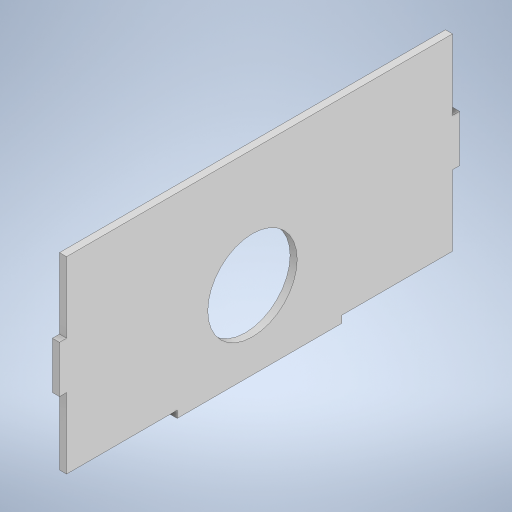
# Autodesk Inventor part: Kanan Kipas
Saved by Autodesk Inventor 2024 (Build 280153000, 153)
## iProperties
Created: 2023-08-09
Part Number: Kanan Kipas
Material: Generic
Document SubType Name: Modeling
Designer: Asus
Density: 1 g/cm^3
Appearance: Default
Author: Asus
Autodesk Inventor part; units mm, degrees
ref_plane "YZ Plane" through (0, 0, 0) normal (1, 0, 0) x (0, 1, 0)
ref_plane "XZ Plane" through (0, 0, 0) normal (0, 1, 0) x (-1, 0, 0)
ref_plane "XY Plane" through (0, 0, 0) normal (0, 0, 1) x (1, 0, 0)
sketch "Sketch2" plane through (0, 0, 0) normal (1, 0, 0) x (0, 1, 0)
  line L0 (0, 0) -> (3, 0) construction
  line L1 (3, 0) -> (3, -3)
  line L2 (3, -3) -> (3, -50)
  line L3 (3, -50) -> (0, -50)
  line L4 (0, -50) -> (0, -120)
  line L5 (0, -120) -> (3, -120)
  line L6 (3, -120) -> (3, -170)
  line L7 (33, -170) -> (33, -167)
  line L8 (53, -167) -> (53, -170)
  line L9 (53, 0) -> (53, -3)
  line L10 (33, -3) -> (33, 0)
  line L11 (0, 0) -> (0, -63) construction
  line L12 (0, -63) -> (14, -63) construction
  line L13 (14, -63) -> (14, -82) construction
  line L14 (14, -82) -> (33, -82) construction
  circle A0 centre (33, -82) radius 19
  line L15 (33, -167) -> (3, -167)
  line L16 (53, -167) -> (83, -167)
  line L17 (83, -167) -> (83, -120)
  line L18 (33, -170) -> (53, -170)
  line L19 (53, -3) -> (83, -3)
  line L20 (33, -3) -> (3, -3)
  line L21 (33, 0) -> (53, 0)
  line L22 (83, -3) -> (83, -120)
  dimension "d0" = 3
  dimension "d1" = 3
  dimension "d2" = 47
  dimension "d3" = 70
  dimension "d4" = 50
  dimension "d5" = 30
  dimension "d6" = 3
  dimension "d7" = 20
  dimension "d11" = 3
  dimension "d12" = 20
  dimension "d15" = 63
  dimension "d16" = 14
  dimension "d19" = 19
  dimension "d20" = 19
  dimension "d21" = 30
  dimension "d22" = 170
  constraints: 46 end point, 6 point on line, 5 perpendicular, 2 collinear, 2 horizontal, 2 vertical, 1 centre point, 1 coincident, 1 parallel
  measures "d0" distance of L0.start L0.end
  measures "d1" distance of L0.end L1.end
  measures "d2" distance of L1.end L2.end
  measures "d3" distance of L3.end L4.end
  measures "d4" distance of L5.end L6.end
  measures "d5" distance of L6.end L7.start
  measures "d6" distance of L7.start L7.end
  measures "d7" distance of L7.end L8.start
  measures "d11" distance of L9.start L9.end
  measures "d12" distance of L9.end L10.start
  measures "d15" distance of L0.start L11.end
  measures "d16" distance of L11.end L12.end
  measures "d19" distance of L12.end L13.end
  measures "d20" distance of L13.end L14.end
  measures "d21" distance of L8.start L16.end
  measures "d22" distance between parallel lines of L18 L21
extrude "Extrusion1" add sketch "Sketch2" along normal blind 3
body "Solid1"
